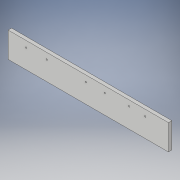
# Autodesk Inventor part: Kermit bumper 2 large ( middle not finished yet)
Saved by Autodesk Inventor 2018.2 (Build 222227000, 227)
## iProperties
Created: 2018-02-13
Part Number: Kermit bumper 2 large ( middle not finished yet)
Material: Generic
Document SubType Name: Modeling
Designer: kalra.rohan
Density: 1 g/cm^3
Appearance: Default
Author: kalra.rohan
Autodesk Inventor part; units mm, degrees
ref_plane "YZ Plane" through (0, 0, 0) normal (1, 0, 0) x (0, 1, 0)
ref_plane "XZ Plane" through (0, 0, 0) normal (0, 1, 0) x (-1, 0, 0)
ref_plane "XY Plane" through (0, 0, 0) normal (0, 0, 1) x (1, 0, 0)
sketch "Sketch1" plane through (0, 0, 0) normal (0, 0, 1) x (1, 0, 0)
  line L0 (0, 0) -> (882.65, 0)
  line L1 (882.65, 0) -> (882.65, -139.7)
  line L2 (882.65, -139.7) -> (0, -139.7)
  line L3 (0, -139.7) -> (0, 0)
  circle A0 centre (754.4805, -34.29) radius 3.81
  circle A1 centre (665.5805, -30.48) radius 3.81
  circle A2 centre (532.2305, -34.29) radius 3.81
  circle A3 centre (428.0905, -34.29) radius 3.81
  circle A4 centre (212.1905, -34.29) radius 3.81
  circle A5 centre (99.2611, -34.29) radius 3.81
  dimension "d0" = 882.65
  dimension "d1" = 139.7
  dimension "d2" = 7.62
  dimension "d4" = 7.62
  dimension "d6" = 7.62
  dimension "d8" = 7.62
  dimension "d9" = 104.14
  dimension "d10" = 7.62
  dimension "d11" = 215.9
  dimension "d12" = 7.62
  dimension "d16" = 105.41
  dimension "d17" = 105.41
  dimension "d18" = 105.41
  dimension "d19" = 105.41
  dimension "d21" = 105.41
  dimension "d22" = 105.41
  dimension "d23" = 88.9
  dimension "d24" = 133.35
  constraints: 8 end point, 6 centre point, 2 parallel, 1 horizontal, 1 perpendicular
  measures "d0" distance between parallel lines of L1 L3
  measures "d1" distance between parallel lines of L0 L2
  measures "d2" diameter of A0
  measures "d4" diameter of A1
  measures "d6" diameter of A2
  measures "d8" diameter of A3
  measures "d9" distance of A2.centre A3.centre
  measures "d10" diameter of A4
  measures "d11" distance of A3.centre A4.centre
  measures "d12" diameter of A5
  measures "d16" distance from line of A3.centre L2
  measures "d17" distance from line of A2.centre L2
  measures "d18" distance edge to line of A1 L2
  measures "d19" distance from line of A0.centre L2
  measures "d21" distance from line of L2 A4.centre
  measures "d22" distance from line of L2 A5.centre
  measures "d23" horizontal distance of A0.centre A1.centre
  measures "d24" horizontal distance of A1.centre A2.centre
extrude "Extrusion1" add sketch "Sketch1" against normal blind 19.05
body "Solid1"
